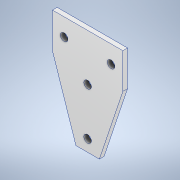
# Autodesk Inventor part: FrameJointT1510
Saved by Autodesk Inventor 2022.3 (Build 263350000, 350)
## iProperties
Created: 2022-04-07
Part Number: FrameJointT1510
Material: アルミニウム 6061
Document SubType Name: Modeling
Designer: satot
Density: 2.7 g/cm^3
Appearance: アルミニウム - フラット
Author: satot
Autodesk Inventor part; units mm, degrees
ref_plane "YZ Plane" through (0, 0, 0) normal (1, 0, 0) x (0, 1, 0)
ref_plane "XZ Plane" through (0, 0, 0) normal (0, 1, 0) x (-1, 0, 0)
ref_plane "XY Plane" through (0, 0, 0) normal (0, 0, 1) x (1, 0, 0)
sketch "スケッチ1" plane through (0, 0, 0) normal (1, 0, 0) x (0, 1, 0)
  line L0 (-5, 30) -> (5, 30)
  line L1 (5, 30) -> (5, 0)
  line L2 (5, 0) -> (-5, 0)
  line L3 (-5, 0) -> (-5, 30)
  line L4 (-15, 45) -> (15, 45)
  line L5 (15, 45) -> (15, 30)
  line L6 (15, 30) -> (-15, 30)
  line L7 (-15, 30) -> (-15, 45)
  line L8 (15, 30) -> (5, 0)
  line L9 (-5, 0) -> (-15, 30)
  point P0 (0, 0)
  point P1 (0, 0)
  point P2 (0, 30)
  dimension "d0" = 10
  dimension "d1" = 30
  dimension "d2" = 30
  dimension "d3" = 15
  constraints: 20 end point, 4 parallel, 3 midpoint, 2 horizontal, 2 perpendicular, 1 coincident
  measures "d0" distance of L1.end L2.end
  measures "d1" distance of L0.end L1.end
  measures "d2" distance of L5.end L6.end
  measures "d3" distance of L4.end L5.end
extrude "押し出し1" add sketch "スケッチ1" along normal blind 2
sketch "スケッチ2" plane through (2, 0, 0) normal (1, 0, 0) x (0, 0, -1)
  line L0 (0, -5) -> (0, 5) projected
  line L1 (-30, 15) -> (-45, 15) projected
  line L2 (-45, -15) -> (-30, -15) projected
  point P0 (0, 0)
  point P1 (-37.5, 10)
  point P2 (-37.5, -10)
  point P3 (-25, 0)
  point P4 (-5, 0)
  point P5 (0, 0)
  point P6 (-37.5, 15)
  dimension "d6" = 5
  dimension "d7" = 20
  dimension "d8" = 5
  dimension "d9" = 5
  constraints: 2 horizontal alignment, 2 midpoint, 2 vertical alignment
  measures "d6" distance from line of L0 point (-5, 0)
  measures "d7" distance of point (-25, 0) point (-5, 0)
  measures "d8" distance from line of L1 point (-37.5, 10)
  measures "d9" distance from line of L2 point (-37.5, -10)
hole "穴1" at (2, 10, 37.5) at (2, -10, 37.5) at (2, 0, 25) at (2, 0, 5) direction (-1, 0, 0) diameter 3.2 end through all
